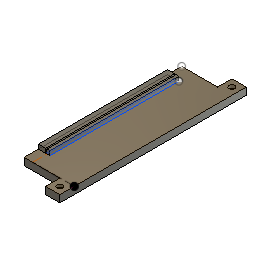
light box cover v3 (Autodesk Fusion 360 design; units mm, degrees)
Autodesk Fusion 360 part; units mm, degrees
sketch "cover base" plane through (0, 0, 0) normal (0, 1, 0) x (1, 0, 0)
  line L0 (17.5, -55) -> (-17.5, -55)
  line L1 (-17.5, -55) -> (-17.5, 55)
  line L2 (-17.5, 55) -> (17.5, 55)
  line L3 (17.5, 55) -> (17.5, -55)
  line L4 (17.5, -55) -> (-17.5, 55) construction
  line L5 (-17.5, -55) -> (17.5, 55) construction
  dimension "d1" = 35
  dimension "d2" = 110
extrude "Extrude1" add sketch "cover base" along normal blind 5
sketch "Screw holder" plane through (0, 0, 0) normal (0, -1, 0) x (1, 0, 0)
  line L0 (-17.5, -55) -> (17.5, -55)
  line L1 (17.5, -55) -> (17.5, 55)
  line L2 (17.5, 55) -> (-17.5, 55)
  line L3 (-17.5, 55) -> (-17.5, -55)
  line L4 (7.5, 55) -> (17.5, 55)
  line L5 (17.5, 55) -> (17.5, 65)
  line L6 (17.5, 65) -> (7.5, 65)
  line L7 (7.5, 65) -> (7.5, 55)
  circle A0 centre (12.5, 60) radius 4
  circle A1 centre (12.5, 60) radius 2
  dimension "d5" = 10
  dimension "d6" = 10
  dimension "d9" = 8
  dimension "d10" = 4
  measures "d9" diameter of A0
  measures "d10" diameter of A1
extrude "Extrude2" add sketch "Screw holder" against normal blind 5 contours L2 L4 L5 L6 L7 | A0 | A1
extrude "Extrude3" cut sketch "Screw holder" against normal up to surface (5 mm away) contours A1
extrude "Extrude4" cut sketch "Screw holder" against normal blind 3 contours A0
mirror "Mirror1" about plane through (0, 0, 0) normal (0, 0, 1) of "Extrude2", "Extrude3", "Extrude4"
sketch "Slit" plane through (0, 5, 0) normal (0, 1, 0) x (-1, 0, 0)
  circle A0 centre (-12.5, -60) radius 2
  circle A1 centre (-12.5, 60) radius 2
  line L0 (-7.5, -55) -> (17.5, -55)
  line L1 (17.5, -55) -> (17.5, 55)
  line L2 (17.5, 55) -> (-7.5, 55)
  line L3 (-7.5, 55) -> (-7.5, 65)
  line L4 (-7.5, 65) -> (-17.5, 65)
  line L5 (-17.5, 65) -> (-17.5, -65)
  line L6 (-17.5, -65) -> (-7.5, -65)
  line L7 (-7.5, -65) -> (-7.5, -55)
  line L8 (-17.5, 55) -> (11.5, 55) construction
  line L9 (17.5, 45) -> (9.5, 45)
  line L10 (9.5, 45) -> (9.5, -45)
  line L11 (9.5, -45) -> (17.5, -45)
  line L12 (17.5, -45) -> (17.5, 45)
  line L13 (11.5, 55) -> (11.5, 45) construction
  line L14 (12.5, 45) -> (11.5, 45)
  line L15 (11.5, 45) -> (11.5, -45)
  line L16 (11.5, -45) -> (12.5, -45)
  line L17 (12.5, -45) -> (12.5, 45)
  dimension "d16" = 29
  dimension "d23" = 8
  dimension "d35" = 90
  dimension "d36" = 90
  dimension "d37" = 1
extrude "Extrude5" add sketch "Slit" along normal blind 3 contours L1 L9 L11 L12 L17 | L9 L11 L14 L15 L16 L17 | L9 L10 L11 L15
extrude "Extrude8" cut sketch "Slit" along normal blind 3 contours L9 L11 L14 L15 L16 L17
fillet "Fillet1" [suppressed]
fillet "Fillet2" [suppressed]
fillet "Fillet3" [suppressed]
sketch "Sketch5" plane through (0, 0, 0) normal (0, -1, 0) x (1, 0, 0)
  line L0 (-16.5, 55) -> (-16.5, -55)
  line L1 (-16.5, -55) -> (5.5, -55)
  arc A0 (7.5, -57) -> (5.5, -55) centre (5.5, -57) ccw
  line L2 (7.5, -57) -> (7.5, -65)
  line L3 (7.5, -65) -> (17.5, -65)
  line L4 (17.5, -65) -> (17.5, 65)
  line L5 (17.5, 65) -> (7.5, 65)
  line L6 (7.5, 65) -> (7.5, 57)
  arc A1 (5.5, 55) -> (7.5, 57) centre (5.5, 57) ccw
  line L7 (5.5, 55) -> (-16.5, 55)
  circle A2 centre (12.5, -60) radius 4
  circle A3 centre (12.5, 60) radius 4
  line L8 (12.5, -60) -> (12.5, -45) construction
  circle A4 centre (12.5, -45) radius 3
  dimension "d29" = 15
  dimension "d30" = 6
  measures "d30" diameter of A4
extrude "Extrude7" [suppressed]
